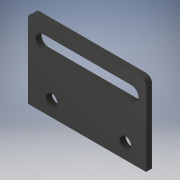
# Autodesk Inventor part: Radio Chip
Saved by Autodesk Inventor 2019 (Build 230136000, 136)
## iProperties
Created: 2019-10-24
Part Number: Radio Chip
Material: UHMW, Black
Document SubType Name: Modeling
Designer: robgr
Density: 0.94 g/cm^3
Appearance: Smooth - Black
Mass: 1.66101 g
Surface Area: 22.3328 cm^2
Volume: 1.76703 cm^3
Author: robgr
Autodesk Inventor part; units mm, degrees
ref_plane "YZ Plane" through (0, 0, 0) normal (1, 0, 0) x (0, 1, 0)
ref_plane "XZ Plane" through (0, 0, 0) normal (0, 1, 0) x (-1, 0, 0)
ref_plane "XY Plane" through (0, 0, 0) normal (0, 0, 1) x (1, 0, 0)
sketch "Sketch1" plane through (0, 0, 0) normal (0, 0, 1) x (1, 0, 0)
  line L0 (-22.0668, 11.5486) -> (13.9332, 11.5486)
  line L1 (15.9332, 9.5486) -> (15.9332, -15.4514)
  line L2 (15.9332, -15.4514) -> (-24.0668, -15.4514)
  line L3 (-24.0668, -15.4514) -> (-24.0668, 9.5486)
  circle A0 centre (-16.0668, -10.4514) radius 2
  circle A1 centre (8.9332, -10.4514) radius 2
  arc A2 (-22.0668, 11.5486) -> (-24.0668, 9.5486) centre (-22.0668, 9.5486) ccw
  arc A3 (15.9332, 9.5486) -> (13.9332, 11.5486) centre (13.9332, 9.5486) ccw
  line L4 (10.9332, 5.0486) -> (-19.0668, 5.0486) construction
  line L5 (10.9332, 7.5486) -> (-19.0668, 7.5486)
  line L6 (-19.0668, 2.5486) -> (10.9332, 2.5486)
  arc A4 (10.9332, 2.5486) -> (10.9332, 7.5486) centre (10.9332, 5.0486) ccw
  arc A5 (-19.0668, 7.5486) -> (-19.0668, 2.5486) centre (-19.0668, 5.0486) ccw
  point P0 (0, 0)
  point P1 (-4.0668, 5.0486)
  dimension "d0" = 40
  dimension "d1" = 4
  dimension "d2" = 4
  dimension "d3" = 25
  dimension "d4" = 8
  dimension "d5" = 2
  dimension "d6" = 5
  dimension "d7" = 15
  dimension "d8" = 5
  dimension "d11" = 25
  dimension "d12" = 4
  constraints: 16 end point, 8 point on circle, 8 tangent, 6 centre point, 3 parallel, 2 horizontal, 1 equal radius, 1 midpoint, 1 perpendicular
  measures "d0" distance of L1.end L2.end
  measures "d1" diameter of A0
  measures "d2" diameter of A1
  measures "d3" distance of A1.centre A0.centre
  measures "d4" distance from line of L3 A0.centre
  measures "d5" radius of A2
  measures "d6" distance from line of L2 A0.centre
  measures "d7" distance of point (-4.067, 5.049) L4.end
  measures "d8" diameter of A5
  measures "d11" distance of L2.end L3.end
  measures "d12" distance between parallel lines of L0 L5
extrude "Extrusion1" add sketch "Sketch1" along normal blind 2
body "Solid1"
